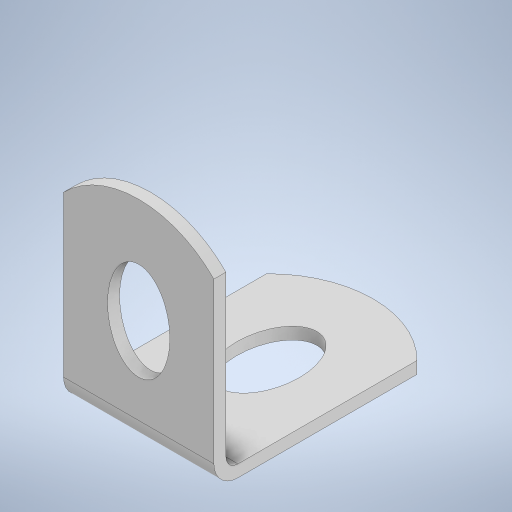
# Autodesk Inventor part: Уголок
Saved by Autodesk Inventor 2023.2 (Build 272271030, 271C)
## iProperties
Created: 2024-03-27
Part Number: Уголок
Material: Типовые
Document SubType Name: Sheet Metal
Designer: I9232
Density: 1 g/cm^3
Sheet Metal Rule: По умолчанию
Appearance: По умолчанию
Author: I9232
Autodesk Inventor part; units mm, degrees
ref_plane "YZ Plane" through (0, 0, 0) normal (1, 0, 0) x (0, 1, 0)
ref_plane "XZ Plane" through (0, 0, 0) normal (0, 1, 0) x (-1, 0, 0)
ref_plane "XY Plane" through (0, 0, 0) normal (0, 0, 1) x (1, 0, 0)
sketch "Эскиз1" plane through (0, 0, 0) normal (0, 1, 0) x (-1, 0, 0)
  line L0 (5, -14) -> (-5, -14)
  line L1 (-5, -14) -> (-5, 0)
  line L2 (-5, 0) -> (5, 0)
  line L3 (5, 0) -> (5, -14)
  line L4 (0, -10.25) -> (0, -3.75)
  line L5 (0, -14) -> (0, 0) construction
  ellipse E0 centre (0, -7) end of major axis (-2.075, -7) minor radius 3.25
  dimension "d5" = 2.075
  dimension "d0" = 14
  dimension "d1" = 10
  dimension "d4" = 6.5
  constraints: 12 end point, 4 midpoint, 3 coincident, 3 vertical, 2 parallel, 1 horizontal, 1 perpendicular, 1 vertical alignment, 2 other
  measures "d0" distance of L0.end L1.end
  measures "d1" distance of L0.start L0.end
  measures "d4" distance of L4.start L4.end
extrude "Выдавливание1" add sketch "Эскиз1" along normal mid plane 0.8
mirror "Зеркальное отражение1" about plane through (0, 0, 0) normal (0, 0, 1) of "Выдавливание1"
sketch "Эскиз2" plane through (0, 0.4, 0) normal (0, 1, 0) x (1, 0, 0)
  point P0 (0, 0)
sketch "Эскиз3" plane through (0, 0.4, 0) normal (0, 1, 0) x (1, 0, 0)
  ellipse E0 centre (0, 7) end of major axis (0, 10.25) minor radius 2.075 projected
  line L0 (5, 14) -> (-5, 14) projected
  arc A0 (5, 11.899) -> (0, 14) centre (0, 7) ccw
  arc A1 (0, 14) -> (-5, 11.899) centre (0, 7) ccw
  line L1 (5, 14) -> (5, -14) projected
  line L2 (-5, 14) -> (-5, -14) projected
  line L3 (2.799, 0) -> (-2.799, 0) construction
  arc A2 (0, -14) -> (5, -11.899) centre (0, -7) ccw
  arc A3 (-5, -11.899) -> (0, -14) centre (0, -7) ccw
  line L4 (5, -14) -> (-5, -14) projected
  point P0 (0, 0)
  point P1 (0, 0)
  point P2 (5, -11.899)
  constraints: 8 point on circle, 5 symmetric about line, 4 centre point, 4 coincident, 2 end point, 2 midpoint, 2 point on line, 1 horizontal, 3 other
extrude "Выдавливание2" cut sketch "Эскиз3" against normal up to surface (0.8 mm away) contours L1 A0 L0 | A1 L2 L0 | L1 L4 A2 | A3 L4 L2
sketch "Эскиз5" plane through (0, 0.4, 0) normal (0, 1, 0) x (1, 0, 0)
  line L0 (-5, 11.899) -> (-5, -11.899) projected
  line L1 (-5, 0) -> (5, 0)
  line L2 (5, 11.899) -> (5, -11.899) projected
  point P0 (0, 0)
  constraints: 2 end point, 2 midpoint
bend part "Сгиб детали1" radius 0.8 angle 90 line through (-5, 0.4, 0) along (1, 0, 0) centre toward (0, 1, 0) moving side (0, 0, 1) both sides no
equation "\"Радиус_гибки\" = Толщина"
equation "\"Ширина_просечки\" = Толщина"
equation "\"Глубина_просечки\" = 0.5 * Толщина"
equation "\"Размер_просечки\" = 4 * Толщина"
equation "\"Мин_остаток\" = 2 * Толщина"
equation "\"Радиус_перехода\" = Радиус_гибки"
equation "\"Радиус_Якоби\" = Радиус_гибки"
equation "\"Размер_зазора\" = Толщина"
equation "\"Толщина\" = 0.8"
